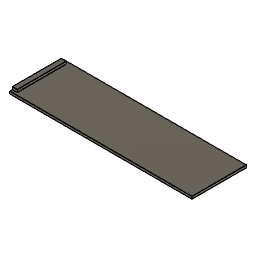
Canal - top plate v2 (Autodesk Fusion 360 design; units mm, degrees)
Autodesk Fusion 360 part; units mm, degrees
sketch "Esquisse1" plane through (0, 0, 0) normal (0, 0, 1) x (1, 0, 0)
  line L0 (-5.6946, 30) -> (67.3054, 30)
  line L1 (67.3054, 30) -> (67.3054, 8.2)
  line L2 (67.3054, 8.2) -> (-5.6946, 8.2)
  line L3 (-5.6946, 8.2) -> (-5.6946, 30)
  dimension "d1" = 73
  dimension "d2" = 21.8
  constraint horizontal L0
  constraint vertical L1
  constraint horizontal L2
  constraint vertical L3
  measures "d1" distance of L1 L3
  measures "d2" distance of L0 L2
extrude "Extrusion1" add sketch "Esquisse1" along normal blind 1
sketch "Esquisse2" plane through (0, 0, 1) normal (0, 0, 1) x (-1, 0, 0)
  line L0 (5.6946, -8.2) -> (-67.3054, -8.2)
  line L1 (-67.3054, -8.2) -> (-67.3054, -30)
  line L2 (-67.3054, -30) -> (5.6946, -30)
  line L3 (5.6946, -30) -> (5.6946, -8.2)
  line L4 (5.6946, -9.3) -> (3.6946, -9.3)
  line L5 (3.6946, -9.3) -> (3.6946, -28.9)
  line L6 (3.6946, -28.9) -> (5.6946, -28.9)
  line L7 (5.6946, -28.9) -> (5.6946, -9.3)
  line L8 (-67.3054, -19.1) -> (5.6946, -19.1) construction
  dimension "d5" = 19.6
  dimension "d8" = 2
  constraint horizontal L4
  constraint vertical L5
  constraint horizontal L6
  constraint vertical L7
  constraint coincident L3 L4.start
  constraint midpoint L1 L8.start
  constraint midpoint L3 L8.end
  constraint symmetric L4 L6 L8
  measures "d5" distance of L4.end L5.end
  measures "d8" distance of L5.end L6.end
extrude "Extrusion2" add sketch "Esquisse2" along normal blind 1 contours L3 L4 L5 L6 L7
equation "d8 = DesignConfigurationRule.64bc9023-8e4e-4cc4-8a85-19370bf7f1c2.dsgcfgrule"
